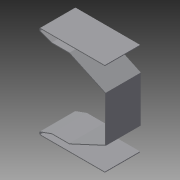
# Autodesk Inventor part: Garra
Saved by Autodesk Inventor 2015 (Build 190159000, 159)
## iProperties
Created: 2016-08-21
Part Number: Garra
Material: Genérico
Document SubType Name: Chapa
Designer: Rodrigo
Density: 1 g/cm^3
Sheet Metal Rule: Padrão_mm
Appearance: Padrão
Author: Rodrigo
Autodesk Inventor part; units mm, degrees
ref_plane "YZ Plane" through (0, 0, 0) normal (1, 0, 0) x (0, 1, 0)
ref_plane "XZ Plane" through (0, 0, 0) normal (0, 1, 0) x (-1, 0, 0)
ref_plane "XY Plane" through (0, 0, 0) normal (0, 0, 1) x (1, 0, 0)
sketch "Esboço1" plane through (0, 0, 0) normal (0, 1, 0) x (-1, 0, 0)
  circle A0 centre (0, 0) radius 40
  line L0 (-40, 0) -> (-40, -25.4828)
  line L1 (-40, -25.4828) -> (0.3313, -44.2896)
  line L2 (0.3313, -44.2896) -> (19.9786, -44.2896)
  line L3 (20.6627, -44.4102) -> (33.3415, -49.0249)
  line L4 (32.6574, -52.9043) -> (-40, -52.9043)
  arc A1 (32.6574, -52.9043) -> (33.3415, -49.0249) centre (32.6574, -50.9043) ccw
  arc A2 (20.6627, -44.4102) -> (19.9786, -44.2896) centre (19.9786, -46.2896) ccw
  line L5 (-40, -52) -> (32.6574, -52)
  arc A3 (32.6574, -52) -> (33.0322, -49.8747) centre (32.6574, -50.9043) ccw
  line L6 (33.0322, -49.8747) -> (20.3534, -45.26)
  arc A4 (20.3534, -45.26) -> (19.9786, -45.1939) centre (19.9786, -46.2896) ccw
  line L7 (19.9786, -45.1939) -> (0.1308, -45.1939)
  line L8 (0.1308, -45.1939) -> (-40.9043, -26.0589)
  line L9 (-40.9043, -26.0589) -> (-40.9043, 0)
  line L10 (-40, -52) -> (-40, -52.9043)
  line L11 (40, 0) -> (-40, 0)
  line L12 (-40, 0) -> (-40, 25.4828)
  line L13 (-40, 25.4828) -> (0.3313, 44.2896)
  line L14 (0.3313, 44.2896) -> (19.9786, 44.2896)
  line L15 (20.6627, 44.4102) -> (33.3415, 49.0249)
  line L16 (32.6574, 52.9043) -> (-40, 52.9043)
  arc A5 (33.3415, 49.0249) -> (32.6574, 52.9043) centre (32.6574, 50.9043) ccw
  arc A6 (19.9786, 44.2896) -> (20.6627, 44.4102) centre (19.9786, 46.2896) ccw
  line L17 (-40, 52) -> (32.6574, 52)
  arc A7 (33.0322, 49.8747) -> (32.6574, 52) centre (32.6574, 50.9043) ccw
  line L18 (33.0322, 49.8747) -> (20.3534, 45.26)
  arc A8 (19.9786, 45.1939) -> (20.3534, 45.26) centre (19.9786, 46.2896) ccw
  line L19 (19.9786, 45.1939) -> (0.1308, 45.1939)
  line L20 (0.1308, 45.1939) -> (-40.9043, 26.0589)
  line L21 (-40.9043, 26.0589) -> (-40.9043, 0)
  line L22 (-40, 52) -> (-40, 52.9043)
  point P0 (20.3313, -44.2896)
  dimension "d0" = 80
  dimension "d1" = 115
  dimension "d4" = 20
  dimension "d5" = 160
  dimension "d6" = 2
  dimension "d7" = 0.9043
  dimension "d8" = 7.7104
  dimension "d9" = 34.6649
  dimension "d10" = 20.6748
  constraints: 46 end point, 18 point on circle, 16 symmetric about line, 9 centre point, 7 tangent, 2 horizontal, 2 parallel, 2 point on line, 1 coincident, 1 equal radius, 1 perpendicular, 1 vertical, 10 other
  measures "d0" diameter of A0
  measures "d1" angle of L1 L0
  measures "d4" distance of L1.end point (20.331, -44.29)
  measures "d5" angle of L2 L3
  measures "d6" radius of A1
  measures "d7" distance between parallel lines of L4 L5
  measures "d8" distance between parallel lines of L5 L2
  measures "d9" distance from line of point (0, 0) L3
  measures "d10" distance from line of L9.end L3
extrude "Extrusão1" add sketch "Esboço1" along normal blind 40 contours L13 L12 L0 L1 L2 A2 L3 A1 L4 L10 L5 A3 L6 A4 L7 L8 L9 L21 L20 L19 A8 L18 A7 L17 L22 L16 A5 L15 A6 L14
equation "\"Raio_dobra\" = Espessura"
equation "\"Largura_alívio_de_dobra\" = Espessura"
equation "\"Profundidade_alívio_de_dobra\" = 0.5 * Espessura"
equation "\"Tamanho_alívio_de_dobra\" = 4 * Espessura"
equation "\"Remanescente_mínimo\" = 2 * Espessura"
equation "\"Raiodetransição\" = Raio_dobra"
equation "\"Tamanho_de_raio_de_Jacobi\" = Raio_dobra"
equation "\"TamanhoFolga\" = Espessura"
equation "\"Espessura\" = 0.5"
